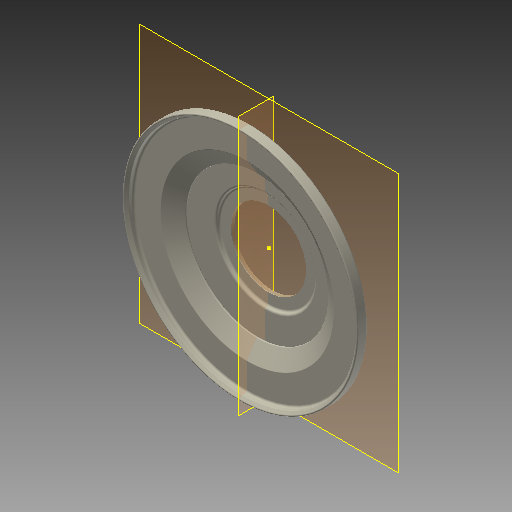
# Autodesk Inventor part: MBS HEAD CONE SHORT
Saved by Autodesk Inventor 2018.3 (Build 223284000, 284)
## iProperties
Created: 2015-01-15
Material: NYLON 6/6
Vendor: HHMI: JFRC - ID&F
Document SubType Name: Modeling
Designer: ARNOLDJ
Density: 1.13 g/cm^3
Appearance: Beige (PC)
Part Number: MBS HEAD CONE SHORT
RuleStatus: InUse
AfterDocSave0: file://Part Number Cleaner
DESIGN DEPARTMENT: HHMI: JFRC - ID&F
ALTERED ITEM PART NUMBER: N/A
ALTERED ITEM VENDOR: N/A
ALTERED ITEM DESCRIPTION: N/A
Revision Number: 0
Autodesk Inventor part; units mm, degrees
ref_plane "XZ Plane" through (0, 0, 0) normal (0, 1, 0) x (-1, 0, 0)
sketch "Block1" plane through (0, 0, 0) normal (0, 0, 1) x (1, 0, 0)
  arc A0 (3.9831, 9.4624) -> (-4.688, 6.6976) centre (2.611, -1.214) ccw
  arc A1 (-5.469, 6.6348) -> (-4.688, 6.6976) centre (-5.1186, 7.1643) ccw
  line L0 (-5.469, 6.6348) -> (-6.1216, 7.0667)
  arc A2 (-4.699, 4.4191) -> (-6.1216, 7.0667) centre (-7.874, 4.4191) ccw
  line L1 (-4.699, 4.4191) -> (-4.699, -1.0472)
  arc A3 (-4.699, -1.0472) -> (-4.6537, -1.2274) centre (-4.318, -1.0472) ccw
  line L2 (-4.6537, -1.2274) -> (-2.0128, -6.1491)
  arc A4 (-2.0128, -6.1491) -> (-1.6771, -6.35) centre (-1.6771, -5.969) ccw
  line L3 (-1.6771, -6.35) -> (-1.27, -6.35)
  arc A5 (-1.27, -6.35) -> (-0.889, -5.969) centre (-1.27, -5.969) ccw
  line L4 (-0.889, -5.969) -> (-0.889, 1.27)
  arc A6 (0.127, 2.286) -> (-0.889, 1.27) centre (0.127, 1.27) ccw
  line L5 (0.127, 2.286) -> (3.9052, 2.286)
  arc A7 (3.9052, 2.286) -> (4.699, 3.0797) centre (3.9052, 3.0798) ccw
  line L6 (4.699, 3.0797) -> (4.699, 10.0922)
  arc A8 (3.9831, 9.4624) -> (4.699, 10.0922) centre (4.064, 10.0922) ccw
  circle A9 centre (-2.921, 1.0414) radius 0.8255
  circle A10 centre (-2.1082, 6.7056) radius 0.8255
  circle A11 centre (2.1082, 6.7056) radius 0.8255
  circle A12 centre (0, 4.7752) radius 0.8255
  circle A13 centre (2.7432, 3.9116) radius 0.8255
  circle A14 centre (-2.7432, 3.9116) radius 0.8255
  point P0 (-1.106, 2.0087)
sketch "Block2" plane through (0, 0, 0) normal (0, 0, 1) x (1, 0, 0)
  arc A0 (2.088, 10.5598) -> (-7.8347, 7.3814) centre (0, 0) ccw
  arc A1 (-7.31, 5.6331) -> (-7.8347, 7.3814) centre (-10.485, 5.6331) ccw
  line L0 (-7.31, 5.6331) -> (-7.31, 0.1668)
  arc A2 (-7.31, 0.1668) -> (-7.2647, -0.0134) centre (-6.929, 0.1668) ccw
  line L1 (-7.2647, -0.0134) -> (-4.6238, -4.9351)
  arc A3 (-4.6238, -4.9351) -> (-4.2881, -5.136) centre (-4.2881, -4.755) ccw
  line L2 (-4.2881, -5.136) -> (-3.881, -5.136)
  arc A4 (-3.881, -5.136) -> (-3.5, -4.755) centre (-3.881, -4.755) ccw
  line L3 (-3.5, -4.755) -> (-3.5, 2.484)
  arc A5 (-2.484, 3.5) -> (-3.5, 2.484) centre (-2.484, 2.484) ccw
  line L4 (-2.484, 3.5) -> (1.2942, 3.5)
  arc A6 (1.2942, 3.5) -> (2.088, 4.2937) centre (1.2942, 4.2937) ccw
  line L5 (2.088, 4.2937) -> (2.088, 10.5598)
  point P0 (-3.6972, 1.0897)
sketch "Block3" plane through (0, 0, 0) normal (0, 0, 1) x (1, 0, 0)
  arc A0 (2.088, 10.5598) -> (-7.8347, 7.3814) centre (0, 0) ccw
  arc A1 (-7.31, 5.6331) -> (-7.8347, 7.3814) centre (-10.485, 5.6331) ccw
  line L0 (-7.3119, 5.6331) -> (-7.3081, 0.1668)
  arc A2 (-7.31, 0.1668) -> (-7.2647, -0.0134) centre (-6.929, 0.1668) ccw
  line L1 (-7.2647, -0.0134) -> (-4.6238, -4.9351)
  arc A3 (-4.6238, -4.9351) -> (-4.2881, -5.136) centre (-4.2881, -4.755) ccw
  line L2 (-4.2881, -5.136) -> (-3.881, -5.136)
  arc A4 (-3.881, -5.136) -> (-3.5, -4.755) centre (-3.881, -4.755) ccw
  line L3 (-3.5, -4.755) -> (-3.5, 2.484)
  arc A5 (-2.484, 3.5) -> (-3.5, 2.484) centre (-2.484, 2.484) ccw
  line L4 (-2.484, 3.5) -> (1.2942, 3.5)
  arc A6 (1.2942, 3.5) -> (2.088, 4.2937) centre (1.2942, 4.2937) ccw
  line L5 (2.088, 4.2937) -> (2.088, 10.5598)
  point P0 (-3.6339, 0.9702)
sketch "Sketch2" plane through (0, 0, 0) normal (0, 0, 1) x (1, 0, 0)
  line L0 (-13.292, 0) -> (6.3572, 0) projected
  line L1 (0, 15.7144) -> (0, -9.0608) projected
  circle A0 centre (0, 0) radius 3.5502 construction
  circle A1 centre (-5.532, 2.2554) radius 0.8255 construction
  circle A2 centre (-4.7192, 7.9196) radius 0.8255 construction
  circle A3 centre (-0.5028, 7.9196) radius 0.8255 construction
  circle A4 centre (-2.611, 5.9892) radius 0.8255 construction
  circle A5 centre (0.1322, 5.1256) radius 0.8255 construction
  circle A6 centre (-5.3542, 5.1256) radius 0.8255 construction
  arc A7 (-7.564, 5.6351) -> (-8.161, 7.4027) centre (-10.485, 5.6331) ccw
  arc A8 (2.342, 10.7664) -> (-8.161, 7.4027) centre (0, 0) ccw
  line L2 (2.342, 10.7664) -> (2.342, 4.2874)
  line L3 (-7.5602, 0) -> (-4.8476, -5.0552)
  line L4 (-4.2881, -5.39) -> (-3.881, -5.39)
  line L5 (-3.246, -4.755) -> (-3.246, 2.484)
  line L6 (-2.484, 3.246) -> (1.3006, 3.246)
  line L7 (-7.564, 5.6351) -> (-7.5602, 0)
  arc A9 (1.3006, 3.246) -> (2.342, 4.2874) centre (1.3006, 4.2874) ccw
  arc A10 (-2.484, 3.246) -> (-3.246, 2.484) centre (-2.484, 2.484) ccw
  arc A11 (-3.881, -5.39) -> (-3.246, -4.755) centre (-3.881, -4.755) ccw
  arc A12 (-4.8476, -5.0552) -> (-4.2881, -5.39) centre (-4.2881, -4.755) ccw
  point P0 (-3.156, 3.246)
  dimension "d21" = 1.016
  dimension "d11" = 0
  dimension "d12" = 0
  dimension "d13" = 0.254
  dimension "d15" = 0.254
  dimension "d16" = 0.254
  dimension "d17" = 0.254
  dimension "d18" = 0.254
  dimension "d19" = 1.0414
  dimension "d20" = 0.762
  dimension "d22" = 0.635
  dimension "d23" = 0.635
  constraints: 13 centre point, 12 end point, 12 point on circle, 8 tangent, 2 horizontal, 2 point on line, 1 vertical, 6 other
  measures "d11" distance from line of A0.centre L0
  measures "d12" distance from line of A0.centre L1
  measures "d19" radius of A9
  measures "d20" radius of A10
  measures "d22" radius of A11
  measures "d23" radius of A12
sketch "Sketch1" plane through (0, 0, 0) normal (0, 1, 0) x (-1, 0, 0)
  line L0 (0, -2.0428) -> (0, 9.59) projected
  line L1 (0, 7.0692) -> (0, 0)
  line L2 (-16.8982, 7.9282) -> (-11.51, 2.54) construction
  line L3 (-11.51, 2.54) -> (0, 2.54) construction
  line L4 (-22.3748, 0) -> (15.9616, 0) projected
  line L5 (-10.5352, 2.6471) -> (-8.741, 1.5041)
  line L6 (-8.741, 1.2899) -> (-10.033, 0.4668)
  line L7 (-10.6775, 2.286) -> (-9.4501, 1.5041)
  line L8 (-9.4501, 1.2899) -> (-10.668, 0.514)
  arc A0 (-8.741, 1.2899) -> (-8.741, 1.5041) centre (-8.8093, 1.397) ccw
  arc A1 (-9.4501, 1.2899) -> (-9.4501, 1.5041) centre (-9.5184, 1.397) ccw
  line L9 (-10.6034, 2.667) -> (-13.6144, 2.667)
  line L10 (-14.3764, 2.667) -> (-14.3764, 2.7741)
  line L11 (-14.3764, 2.286) -> (-14.3764, 3.429)
  line L12 (-14.1596, 3.5188) -> (-13.9056, 3.2648)
  line L13 (-13.8684, 3.175) -> (-13.8684, 2.921)
  arc A2 (-13.8684, 2.921) -> (-13.6144, 2.667) centre (-13.6144, 2.921) ccw
  arc A3 (-14.1596, 3.5188) -> (-14.3764, 3.429) centre (-14.2494, 3.429) ccw
  arc A4 (-13.8684, 3.175) -> (-13.9056, 3.2648) centre (-13.9954, 3.175) ccw
  arc A5 (-10.5352, 2.6471) -> (-10.6034, 2.667) centre (-10.6034, 2.54) ccw
  line L14 (-10.033, 0.4668) -> (-10.033, 0.4572)
  line L15 (-10.668, 0.514) -> (-10.668, 0)
  line L16 (-10.668, 0) -> (-9.906, 0)
  line L17 (-9.906, 0) -> (-6.5024, 0)
  line L18 (-5.9944, 0.4572) -> (-5.9944, 0.0762)
  line L19 (-5.9944, 0.0762) -> (-4.5974, 0.0762)
  line L20 (-4.5974, 0.0762) -> (-4.5974, -0.381)
  line L21 (-4.5974, -0.381) -> (-6.5024, -0.381)
  line L22 (-6.5024, -0.381) -> (-6.5024, 0)
  line L23 (-10.033, 0.4572) -> (-5.9944, 0.4572)
  line L24 (-14.3764, 2.286) -> (-10.6775, 2.286)
  point P0 (-10.5664, 2.667)
  point P1 (-8.5729, 1.397)
  point P2 (-9.282, 1.397)
  dimension "d24" = 135
  dimension "d25" = 23.02
  dimension "d26" = 7.62
  dimension "d27" = 2.54
  dimension "d47" = 21.336
  dimension "d48" = 0.381
  dimension "d49" = 0.381
  dimension "d50" = 0.127
  dimension "d51" = 32.5
  dimension "d56" = 45
  dimension "d57" = 0.254
  dimension "d58" = 0.127
  dimension "d59" = 65
  dimension "d61" = 0.635
  dimension "d79" = 1.397
  dimension "d80" = 21.1328
  dimension "d90" = 0.4572
  dimension "d91" = 0.508
  dimension "d92" = 9.1948
  dimension "d93" = 0.381
  dimension "d94" = 1.905
  dimension "d96" = 0.4572
  dimension "d97" = 0.381
  dimension "d98" = 3.81
  dimension "d99" = 2.667
  dimension "d100" = 0.508
  dimension "d101" = 1.143
  constraints: 46 end point, 12 point on circle, 12 point on line, 12 tangent, 11 perpendicular, 6 centre point, 3 equal radius, 3 horizontal, 2 parallel, 2 vertical
  measures "d24" angle of L3 L2
  measures "d25" diameter of L2.end L0
  measures "d26" distance of L2.start L2.end
  measures "d27" distance between parallel lines of L4 L3
  measures "d47" diameter of L8.end L0
  measures "d48" distance between parallel lines of L5 L7
  measures "d49" distance between parallel lines of L6 L8
  measures "d50" radius of A0
  measures "d51" angle of L4 L8
  measures "d56" angle of L11 L12
  measures "d57" radius of A2
  measures "d58" radius of A3
  measures "d59" angle of L8 L7
  measures "d61" distance between parallel lines of L14 L15
  measures "d79" distance from line of L4 A1.centre
  measures "d80" diameter of point (-10.566, 2.667) L1
  measures "d90" distance of L19.end L20.end
  measures "d91" distance between parallel lines of L22 L18
  measures "d92" diameter of L20 L1
  measures "d93" distance between parallel lines of L21 L17
  measures "d94" distance of L20.end L21.end
  measures "d96" distance between parallel lines of L17 L23
  measures "d97" distance between parallel lines of L24 L9
  measures "d98" distance from line of point (-10.566, 2.667) L11
  measures "d99" distance between parallel lines of L4 L9
  measures "d100" distance between parallel lines of L13 L11
  measures "d101" distance from line of L24 A3.centre
revolve "Revolution1" add sketch "Sketch1" angle 360 about axis through (0, 0, 0) along (0, 0, 1)
sketch "Sketch3" plane through (0, 0, 0) normal (0, 0, 1) x (1, 0, 0)
  point P0 (0, 0)
sketch "Sketch5" plane through (0, 0, 0) normal (0, 0, 1) x (1, 0, 0)
  point P0 (0, 0)
sketch "Sketch7" plane through (0, 0, 0) normal (0, 0, 1) x (1, 0, 0)
  point P0 (0, 0)
fillet "Fillet1" radius 0.127 1 edges at (-10.668, 0, 0.514)
fillet "Fillet2" radius 0.254 3 edges at (-5.9944, 0, 0.4572) (-5.9944, 0, 0.0762) (-6.5024, 0, 0)
fillet "Fillet3" radius 0.254 2 edges at (-14.3764, 0, 2.286) (-10.6775, 0, 2.286)
body "Solid1"
